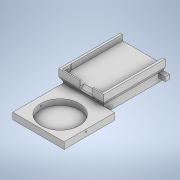
# Autodesk Inventor part: cable_jig_base
Saved by Autodesk Inventor 2022 (Build 260153000, 153)
## iProperties
Created: 2022-03-09
Part Number: cable_jig_base
Material: Generic
Document SubType Name: Modeling
Designer: kylem
Density: 1 g/cm^3
Appearance: Default
Author: kylem
Autodesk Inventor part; units mm, degrees
ref_plane "YZ Plane" through (0, 0, 0) normal (1, 0, 0) x (0, 1, 0)
ref_plane "XZ Plane" through (0, 0, 0) normal (0, 1, 0) x (-1, 0, 0)
ref_plane "XY Plane" through (0, 0, 0) normal (0, 0, 1) x (1, 0, 0)
sketch "Sketch1" plane through (0, 0, 0) normal (0, 1, 0) x (-1, 0, 0)
  line L0 (0, 0) -> (74, 0)
  line L1 (74, 0) -> (74, -140)
  line L2 (74, -140) -> (0, -140)
  line L3 (0, -140) -> (0, 0)
  dimension "d0" = 74
  dimension "d1" = 140
  constraints: 8 end point, 2 parallel, 1 horizontal, 1 perpendicular
  measures "d0" distance of L1.end L2.end
  measures "d1" distance of L0.end L1.end
extrude "Extrusion1" add sketch "Sketch1" along normal blind 25
sketch "Sketch2" plane through (0, 0, 0) normal (0, -1, 0) x (1, 0, 0)
  line L0 (-74, -140) -> (-74, 0) projected
  line L1 (-74, 0) -> (-74, 52.6)
  line L2 (-74, 0) -> (-21.4, 0) construction
  line L3 (-74, 52.6) -> (-27.125, 52.6)
  circle A0 centre (-27.125, 52.6) radius 35.25
  point P0 (0, 0)
  dimension "d4" = 52.6
  dimension "d5" = 90
  dimension "d6" = 46.875
  dimension "d7" = 90
  dimension "d8" = 70.5
  constraints: 6 end point, 2 perpendicular, 1 centre point, 1 coincident, 1 horizontal, 1 vertical
  measures "d4" distance of L0.end L1.end
  measures "d5" angle of L2 L1
  measures "d6" distance of L1.end L3.end
  measures "d7" angle of L1 L3
  measures "d8" diameter of A0
extrude "Extrusion2" add sketch "Sketch2" against normal blind 1.5
sketch "Sketch3" plane through (0, 0, 0) normal (0, -1, 0) x (1, 0, 0)
  line L0 (-74, -140) -> (-74, 0) projected
  line L1 (-74, 0) -> (19.75, 0)
  line L2 (19.75, 0) -> (19.75, 105.2)
  line L3 (19.75, 105.2) -> (-74, 105.2)
  line L4 (-74, 105.2) -> (-74, 0)
  circle A0 centre (-27.125, 52.6) radius 35.25
  point P0 (0, 0)
  dimension "d11" = 93.75
  dimension "d12" = 105.2
  dimension "d13" = 70.5
  constraints: 8 end point, 2 parallel, 1 centre point, 1 coincident, 1 horizontal, 1 perpendicular
  measures "d11" distance of L3.end L2.end
  measures "d12" distance of L2.end L1.end
  measures "d13" diameter of A0
extrude "Extrusion3" add sketch "Sketch3" against normal blind 10
sketch "Sketch7" plane through (0, 25, 0) normal (0, 1, 0) x (1, 0, 0)
  line L0 (-74, 0) -> (0, 0) projected
  line L1 (-74, 140) -> (-74, 0) projected
  line L2 (0, 0) -> (-74, 0)
  line L3 (-74, 0) -> (-74, 140)
  line L4 (-74, 140) -> (0, 140)
  line L5 (0, 140) -> (0, 0)
  line L6 (0, 0) -> (0, 140) projected
  line L7 (0, 0) -> (4, 0)
  line L8 (4, 0) -> (4, 140)
  line L9 (4, 140) -> (0, 140)
  line L10 (0, 140) -> (0, 0)
  line L11 (-74, 0) -> (-78, 0)
  line L12 (-78, 0) -> (-78, 140)
  line L13 (-78, 140) -> (-74, 140)
  line L14 (-74, 140) -> (-74, 0)
  line L15 (-74, 0) -> (-74, -105.2) projected
  line L16 (0, 0) -> (-74, 0)
  line L17 (-74, 0) -> (-74, -4)
  line L18 (-74, -4) -> (0, -4)
  line L19 (0, -4) -> (0, 0)
  line L20 (4, 0) -> (0, 0)
  line L21 (0, 0) -> (0, -4)
  line L22 (0, -4) -> (4, -4)
  line L23 (4, -4) -> (4, 0)
  line L24 (-78, 0) -> (-74, 0)
  line L25 (-74, 0) -> (-74, -4)
  line L26 (-74, -4) -> (-78, -4)
  line L27 (-78, -4) -> (-78, 0)
  dimension "d34" = 4
  dimension "d35" = 140
  dimension "d36" = 4
  dimension "d37" = 140
  dimension "d38" = 4
  constraints: 48 end point, 12 parallel, 6 horizontal, 6 perpendicular, 1 point on line
  measures "d34" distance of L9.end L8.end
  measures "d35" distance of L8.end L7.end
  measures "d36" distance of L12.end L13.end
  measures "d37" distance of L11.end L12.end
  measures "d38" distance of L17.end L16.end
extrude "Extrusion6" add sketch "Sketch7" along normal mid plane 20 contours L11 L12 L13 L1 | L15 L26 L27 L11 | L0 L19 L18 L15 | L5 L9 L8 L7 | L7 L23 L22 L19
sketch "Sketch8" plane through (0, 0, -140) normal (0, 0, -1) x (-1, 0, 0)
  line L0 (87.6184, 44.2414) -> (-7.8377, 44.2414)
  line L1 (-7.8377, 44.2414) -> (-7.8377, -7.0095)
  line L2 (-7.8377, -7.0095) -> (87.6184, -7.0095)
  line L3 (87.6184, -7.0095) -> (87.6184, 44.2414)
  point P0 (0, 0)
  constraints: 8 end point, 2 parallel, 1 horizontal, 1 perpendicular
extrude "Extrusion7" cut sketch "Sketch8" against normal blind 30
sketch "Sketch9" plane through (-74, 0, 105.2) normal (0, 0, 1) x (1, 0, 0)
  line L0 (-5.172, -2.6476) -> (95.2313, -2.6476)
  line L1 (95.2313, -2.6476) -> (95.2313, 16.8527)
  line L2 (95.2313, 16.8527) -> (-5.172, 16.8527)
  line L3 (-5.172, 16.8527) -> (-5.172, -2.6476)
  point P0 (74, 0)
  constraints: 8 end point, 2 parallel, 1 horizontal, 1 perpendicular
extrude "Extrusion8" cut sketch "Sketch9" against normal blind 10
sketch "Sketch10" plane through (0, 25, 0) normal (0, 1, 0) x (1, 0, 0)
  line L0 (-74, 0) -> (0, 0) projected
  line L1 (-74, 0) -> (-73, 0)
  line L2 (-73, 0) -> (-73, 15)
  line L3 (-73, 15) -> (-74, 15)
  line L4 (-74, 15) -> (-74, 0)
  point P0 (-73, 0)
  dimension "d48" = 1
  dimension "d49" = 15
  constraints: 8 end point, 2 parallel, 1 horizontal, 1 perpendicular
  measures "d48" distance of L3.end L2.end
  measures "d49" distance of L2.end L1.end
extrude "Extrusion9" add sketch "Sketch10" along normal blind 10
chamfer "Chamfer8" distance 1 angle 75 1 edges at (-73, 30, -15) measured on face at (-73.5, 30, -15)
chamfer "Chamfer9" distance 1 angle 75 1 edges at (-73, 35, -5.634) measured on face at (-73.5, 35, -5.634)
sketch "Sketch11" plane through (0, 35, 0) normal (0, 1, 0) x (1, 0, 0)
  line L0 (0, 0) -> (-74, 0) projected
  line L1 (0, 0) -> (-16, 0)
  line L2 (-74, 0) -> (-78, -4) projected
  line L3 (-74, 0) -> (-41, 0)
  line L4 (-78, -4) -> (4, -4) projected
  line L5 (-16, 0) -> (-41, 0)
  line L6 (-41, 0) -> (-41, -4)
  line L7 (-41, -4) -> (-16, -4)
  line L8 (-16, -4) -> (-16, 0)
  line L9 (-41, -4) -> (-16, -4)
  line L10 (-16, -4) -> (-16, 3)
  line L11 (-16, 3) -> (-41, 3)
  line L12 (-41, 3) -> (-41, -4)
  dimension "d67" = 16
  dimension "d68" = 33
  dimension "d69" = 25
  dimension "d70" = 7
  constraints: 20 end point, 4 parallel, 3 point on line, 2 horizontal, 2 perpendicular
  measures "d67" distance of L0.start L1.end
  measures "d68" distance of L0.end L3.end
  measures "d69" distance of L11.end L10.end
  measures "d70" distance of L10.end L9.end
extrude "Extrusion10" cut sketch "Sketch11" against normal blind 15 contours L8 L4 L6 L0
chamfer "Chamfer10" distance 5 angle 45 1 edges at (-28.5, 25, 0)
chamfer "Chamfer11" distance 6.9282 angle 30 1 edges at (-78, 15, -53) measured on face at (-78, 15.5, -53)
chamfer "Chamfer12" distance 6.9282 angle 30 1 edges at (-35, 15, 4) measured on face at (-35, 15.5, 4)
chamfer "Chamfer13" distance 6.9282 angle 30 1 edges at (4, 15, -55) measured on face at (4, 15.5, -55)
fillet "Fillet1" radius 2 1 edges at (-28.5, 20, 2.8868)
sketch "Sketch12" plane through (0, 0, -110) normal (0, 0, -1) x (-1, 0, 0)
  line L0 (0, 15) -> (74, 15) projected
  line L1 (0, 15) -> (-12, 15)
  line L2 (-12, 15) -> (-12, 7)
  line L3 (-12, 7) -> (0, 7)
  line L4 (0, 7) -> (0, 15)
  line L5 (-12, 11) -> (-9.5, 11)
  circle A0 centre (-9.5, 11) radius 1.425
  line L6 (0, 0) -> (-19.75, 0) projected
  line L7 (74, 15) -> (74, 0) projected
  line L8 (0, 0) -> (74, 0)
  line L9 (74, 0) -> (0, 0) projected
  line L10 (37, 0) -> (37, -5.7929)
  line L11 (74, 15) -> (86, 15)
  line L12 (86, 15) -> (86, 7)
  line L13 (86, 7) -> (74, 7)
  line L14 (74, 7) -> (74, 15)
  line L15 (86, 11) -> (83.5, 11)
  circle A1 centre (83.5, 11) radius 1.425
  dimension "d86" = 12
  dimension "d87" = 8
  dimension "d88" = 2.5
  dimension "d89" = 2.85
  constraints: 24 end point, 6 symmetric about line, 2 centre point, 2 coincident, 2 horizontal, 2 midpoint, 2 parallel, 2 perpendicular, 1 vertical, 1 other
  measures "d86" distance of L3.end L2.end
  measures "d87" distance of L2.end L1.end
  measures "d88" distance of L5.start L5.end
  measures "d89" diameter of A0
extrude "Extrusion11" add sketch "Sketch12" against normal blind 10
sketch "Sketch13" plane through (-73, 25, 0) normal (0, 0, -1) x (-1, 0, 0)
  line L0 (0, 0) -> (-32, 0) projected
  line L1 (-73, 0) -> (-73, 10) projected
  line L2 (0, 0) -> (-73, 0)
  line L3 (-73, 0) -> (-73, 10)
  line L4 (-73, 10) -> (0, 10)
  line L5 (0, 6.2679) -> (0, 0)
  line L6 (-32, 10) -> (1, 10) projected
  line L7 (0, 10) -> (1, 10)
  line L8 (0, 6.2679) -> (1, 10) projected
  line L9 (1, 10) -> (0, 6.2679)
  point P0 (-73, -25)
  constraints: 12 end point, 2 collinear, 2 parallel, 1 horizontal, 1 perpendicular, 1 point on line
extrude "Extrusion12" cut sketch "Sketch13" against normal blind 2
sketch "Sketch14" plane through (0, 0, -110) normal (0, 0, -1) x (-1, 0, 0)
  line L0 (-12, 15) -> (0, 15) projected
  line L1 (0, 7) -> (-12, 7) projected
  line L2 (0, 15) -> (-12, 15)
  line L3 (-12, 15) -> (-12, 7)
  line L4 (-12, 7) -> (0, 7)
  line L5 (0, 7) -> (0, 15)
  line L6 (86, 7) -> (74, 7) projected
  line L7 (74, 15) -> (86, 15) projected
  line L8 (74, 7) -> (86, 7)
  line L9 (86, 7) -> (86, 15)
  line L10 (86, 15) -> (74, 15)
  line L11 (74, 15) -> (74, 7)
  point P0 (0, 0)
  point P1 (74, 15)
  constraints: 16 end point, 4 parallel, 2 horizontal, 2 perpendicular
extrude "Extrusion13" cut sketch "Sketch14" against normal blind 2
sketch "Sketch16" plane through (0, 10, 0) normal (0, 1, 0) x (1, 0, 0)
  line L0 (0, 0) -> (19.75, 0) projected
  line L1 (-74, 110) -> (-74, -95.2) projected
  line L2 (19.75, 0) -> (-74, 0)
  line L3 (-74, 0) -> (-74, -95.2)
  line L4 (-74, -95.2) -> (19.75, -95.2)
  line L5 (19.75, -95.2) -> (19.75, 0)
  circle A0 centre (-27.125, -52.6) radius 35.25 projected
  circle A1 centre (-27.125, -52.6) radius 35.25
  constraints: 8 end point, 2 parallel, 1 centre point, 1 coincident, 1 horizontal, 1 perpendicular
extrude "Extrusion14" add sketch "Sketch16" along normal blind 2
sketch "Sketch19" plane through (-74, 0, -110) normal (-1, 0, 0) x (0, 0, 1)
  line L0 (205.2, 12) -> (205.2, 0) projected
  line L1 (205.2, 12) -> (162.6, 12)
  line L2 (205.2, 12) -> (110, 12) projected
  line L3 (162.6, 12) -> (162.6, 18)
  line L4 (127.35, 12) -> (197.85, 12) projected
  line L5 (162.6, 12) -> (168.6, 12) construction
  line L6 (162.6, 18) -> (162.6, 8)
  circle A0 centre (162.6, 8) radius 1.425
  point P0 (110, 0)
  dimension "d98" = 42.6
  dimension "d99" = 6
  dimension "d100" = 90
  dimension "d101" = 10
  dimension "d102" = 2.85
  constraints: 8 end point, 2 perpendicular, 2 point on line, 1 centre point, 1 coincident, 1 horizontal
  measures "d98" distance of L0.start L1.end
  measures "d99" distance of L1.end L3.end
  measures "d100" angle of L5 L3
  measures "d101" distance of L3.end L6.end
  measures "d102" diameter of A0
extrude "Extrusion15" cut sketch "Sketch19" against normal blind 200
sketch "Sketch20" plane through (-74, 0, 95.2) normal (0, 0, 1) x (1, 0, 0)
  line L0 (93.75, 0) -> (93.75, 12) projected
  line L1 (0, 0) -> (93.75, 0)
  line L2 (93.75, 0) -> (93.75, 12)
  line L3 (93.75, 12) -> (0, 12)
  line L4 (0, 12) -> (0, 0)
  point P0 (74, 0)
  constraints: 8 end point, 2 parallel, 1 horizontal, 1 perpendicular
extrude "Extrusion16" cut sketch "Sketch20" against normal blind 3
sketch "Sketch21" plane through (0, 0, -110) normal (0, 0, -1) x (-1, 0, 0)
  line L0 (-35.2302, 50.59) -> (96.8306, 50.59)
  line L1 (96.8306, 50.59) -> (96.8306, -5.5574)
  line L2 (96.8306, -5.5574) -> (-35.2302, -5.5574)
  line L3 (-35.2302, -5.5574) -> (-35.2302, 50.59)
  point P0 (0, 0)
  constraints: 8 end point, 2 parallel, 1 horizontal, 1 perpendicular
extrude "Extrusion17" cut sketch "Sketch21" against normal blind 2
body "Solid1"
